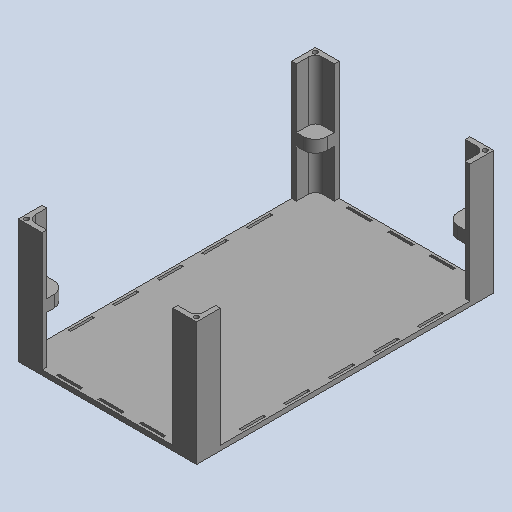
# Autodesk Inventor part: Enclosure_1
Saved by Autodesk Inventor 2026 (Build 300175050, 175E)
## iProperties
Part Number: Enclosure_1
Material: Generic
Document SubType Name: Modeling
Designer: Kartik
Mass: 216.7 g
Surface Area: 1129.54 cm^2
Volume: 216.7 cm^3
Density: 1 g/cm^3
Appearance: Default
Author: Kartik
Autodesk Inventor part; units mm, degrees
ref_plane "YZ Plane" through (0, 0, 0) normal (1, 0, 0) x (0, 1, 0)
ref_plane "XZ Plane" through (0, 0, 0) normal (0, 1, 0) x (-1, 0, 0)
ref_plane "XY Plane" through (0, 0, 0) normal (0, 0, 1) x (1, 0, 0)
sketch "Sketch1" plane through (0, 0, 0) normal (0, 1, 0) x (-1, 0, 0)
  line L0 (31.1634, 169.1828) -> (-118.8366, 169.1828)
  line L1 (-118.8366, 169.1828) -> (-118.8366, -80.8172)
  line L2 (-118.8366, -80.8172) -> (31.1634, -80.8172)
  line L3 (31.1634, -80.8172) -> (31.1634, 169.1828)
  point P0 (0, 0)
  dimension "d0" = 250
  dimension "d1" = 150
  constraints: 8 end point, 2 parallel, 1 horizontal, 1 perpendicular
  measures "d0" distance of L2.end L0.start
  measures "d1" distance of L1.end L2.end
extrude "Extrusion1" add sketch "Sketch1" along normal blind 4
fillet "Fillet1" [suppressed]
sketch "Sketch2" plane through (0, 4, 0) normal (0, 1, 0) x (1, 0, 0)
  line L0 (-31.1634, 80.8172) -> (-31.1634, -169.1828) projected
  line L1 (-31.1634, -169.1828) -> (118.8366, -169.1828) projected
  line L2 (118.8366, -169.1828) -> (118.8366, 80.8172) projected
  line L3 (118.8366, 80.8172) -> (-31.1634, 80.8172) projected
  arc A0 (-21.1634, 76.8172) -> (-27.1634, 70.8172) centre (-21.1634, 70.8172) ccw
  arc A1 (114.8366, 70.8172) -> (108.8366, 76.8172) centre (108.8366, 70.8172) ccw
  arc A2 (108.8366, -165.1828) -> (114.8366, -159.1828) centre (108.8366, -159.1828) ccw
  arc A3 (-27.1634, -159.1828) -> (-21.1634, -165.1828) centre (-21.1634, -159.1828) ccw
  line L4 (108.8366, -165.1828) -> (98.8366, -165.1828)
  line L5 (-11.1634, -165.1828) -> (-21.1634, -165.1828)
  line L6 (-27.1634, -159.1828) -> (-27.1634, -149.1828)
  line L7 (-27.1634, 60.8172) -> (-27.1634, 70.8172)
  line L8 (-21.1634, 76.8172) -> (-11.1634, 76.8172)
  line L9 (98.8366, 76.8172) -> (108.8366, 76.8172)
  line L10 (114.8366, 70.8172) -> (114.8366, 60.8172)
  line L11 (114.8366, -149.1828) -> (114.8366, -159.1828)
  line L12 (-11.1634, -169.1828) -> (-11.1634, -165.1828)
  line L13 (-11.1634, 76.8172) -> (-11.1634, 80.8172)
  line L14 (-31.1634, 60.8172) -> (-27.1634, 60.8172)
  line L15 (114.8366, 60.8172) -> (118.8366, 60.8172)
  line L16 (98.8366, -169.1828) -> (98.8366, -165.1828)
  line L17 (98.8366, 76.8172) -> (98.8366, 80.8172)
  line L18 (-31.1634, -149.1828) -> (-27.1634, -149.1828)
  line L19 (114.8366, -149.1828) -> (118.8366, -149.1828)
  point P0 (0, 0)
  point P1 (114.8366, -154.1828)
  dimension "d12" = 4
  dimension "d13" = 20
  dimension "d14" = 4
  constraints: 32 end point, 8 point on circle, 8 point on line, 4 centre point, 4 vertical, 2 horizontal, 2 perpendicular, 1 midpoint
  measures "d12" distance from line of L2 point (114.837, -154.183)
  measures "d13" distance between parallel lines of L2 L16
  measures "d14" distance between parallel lines of L2 L10
extrude "Extrusion2" add sketch "Sketch2" along normal blind 100 contours L3 L13 L8 A0 L7 L14 L0 | L18 L6 A3 L5 L12 L1 L0 | L3 L2 L15 L10 A1 L9 L17 | L16 L4 A2 L11 L19 L2 L1
sketch "Sketch3" plane through (0, 4, 0) normal (0, 1, 0) x (1, 0, 0)
  line L0 (-29.1634, -129.1828) -> (-27.1634, -129.1828)
  line L1 (-27.1634, -129.1828) -> (-27.1634, -109.1828)
  line L2 (-27.1634, -109.1828) -> (-29.1634, -109.1828)
  line L3 (-29.1634, -109.1828) -> (-29.1634, -129.1828)
  line L4 (-31.1634, 60.8172) -> (-31.1634, -149.1828) projected
  line L5 (-27.1634, -149.1828) -> (-31.1634, -149.1828) projected
  line L6 (-29.1634, -71.6828) -> (-29.1634, -91.6828)
  line L7 (-29.1634, -91.6828) -> (-27.1634, -91.6828)
  line L8 (-27.1634, -91.6828) -> (-27.1634, -71.6828)
  line L9 (-27.1634, -71.6828) -> (-29.1634, -71.6828)
  line L10 (-29.1634, -34.1828) -> (-29.1634, -54.1828)
  line L11 (-29.1634, -54.1828) -> (-27.1634, -54.1828)
  line L12 (-27.1634, -54.1828) -> (-27.1634, -34.1828)
  line L13 (-27.1634, -34.1828) -> (-29.1634, -34.1828)
  line L14 (-29.1634, 3.3172) -> (-29.1634, -16.6828)
  line L15 (-29.1634, -16.6828) -> (-27.1634, -16.6828)
  line L16 (-27.1634, -16.6828) -> (-27.1634, 3.3172)
  line L17 (-27.1634, 3.3172) -> (-29.1634, 3.3172)
  line L18 (-29.1634, 40.8172) -> (-29.1634, 20.8172)
  line L19 (-29.1634, 20.8172) -> (-27.1634, 20.8172)
  line L20 (-27.1634, 20.8172) -> (-27.1634, 40.8172)
  line L21 (-27.1634, 40.8172) -> (-29.1634, 40.8172)
  line L22 (-11.1634, -169.1828) -> (98.8366, -169.1828) projected
  line L23 (114.8366, -129.1828) -> (116.8366, -129.1828)
  line L24 (116.8366, -129.1828) -> (116.8366, -109.1828)
  line L25 (116.8366, -109.1828) -> (114.8366, -109.1828)
  line L26 (114.8366, -109.1828) -> (114.8366, -129.1828)
  line L27 (114.8366, -91.6828) -> (116.8366, -91.6828)
  line L28 (114.8366, -71.6828) -> (114.8366, -91.6828)
  line L29 (116.8366, -71.6828) -> (114.8366, -71.6828)
  line L30 (114.8366, -54.1828) -> (116.8366, -54.1828)
  line L31 (116.8366, -34.1828) -> (114.8366, -34.1828)
  line L32 (114.8366, -34.1828) -> (114.8366, -54.1828)
  line L33 (116.8366, -54.1828) -> (116.8366, -34.1828)
  line L34 (116.8366, -91.6828) -> (116.8366, -71.6828)
  line L35 (114.8366, -16.6828) -> (116.8366, -16.6828)
  line L36 (116.8366, -16.6828) -> (116.8366, 3.3172)
  line L37 (114.8366, 3.3172) -> (114.8366, -16.6828)
  line L38 (116.8366, 3.3172) -> (114.8366, 3.3172)
  line L39 (114.8366, 20.8172) -> (116.8366, 20.8172)
  line L40 (114.8366, 40.8172) -> (114.8366, 20.8172)
  line L41 (116.8366, 40.8172) -> (114.8366, 40.8172)
  line L42 (116.8366, 20.8172) -> (116.8366, 40.8172)
  line L43 (-1.1634, -167.1828) -> (18.8366, -167.1828)
  line L44 (18.8366, -167.1828) -> (18.8366, -165.1828)
  line L45 (18.8366, -165.1828) -> (-1.1634, -165.1828)
  line L46 (-1.1634, -165.1828) -> (-1.1634, -167.1828)
  line L47 (-11.1634, -169.1828) -> (-11.1634, -165.1828) projected
  line L48 (53.8366, -167.1828) -> (53.8366, -165.1828)
  line L49 (53.8366, -165.1828) -> (33.8366, -165.1828)
  line L50 (33.8366, -167.1828) -> (53.8366, -167.1828)
  line L51 (33.8366, -165.1828) -> (33.8366, -167.1828)
  line L52 (88.8366, -167.1828) -> (88.8366, -165.1828)
  line L53 (88.8366, -165.1828) -> (68.8366, -165.1828)
  line L54 (68.8366, -167.1828) -> (88.8366, -167.1828)
  line L55 (68.8366, -165.1828) -> (68.8366, -167.1828)
  line L56 (18.8366, 76.8172) -> (18.8366, 78.8172)
  line L57 (18.8366, 78.8172) -> (-1.1634, 78.8172)
  line L58 (-1.1634, 76.8172) -> (18.8366, 76.8172)
  line L59 (-1.1634, 78.8172) -> (-1.1634, 76.8172)
  line L60 (53.8366, 76.8172) -> (53.8366, 78.8172)
  line L61 (53.8366, 78.8172) -> (33.8366, 78.8172)
  line L62 (33.8366, 76.8172) -> (53.8366, 76.8172)
  line L63 (33.8366, 78.8172) -> (33.8366, 76.8172)
  line L64 (88.8366, 76.8172) -> (88.8366, 78.8172)
  line L65 (88.8366, 78.8172) -> (68.8366, 78.8172)
  line L66 (68.8366, 76.8172) -> (88.8366, 76.8172)
  line L67 (68.8366, 78.8172) -> (68.8366, 76.8172)
  point P0 (0, 0)
  point P1 (-29.1634, -149.1828)
  dimension "d15" = 2
  dimension "d16" = 20
  dimension "d17" = 2
  dimension "d18" = 20
  dimension "d21" = 37.5
  dimension "d28" = 144
  dimension "d33" = 20
  dimension "d34" = 2
  dimension "d35" = 2
  dimension "d36" = 10
  dimension "d39" = 35
  dimension "d42" = 244
  constraints: 128 end point, 4 horizontal, 4 parallel, 2 perpendicular, 2 vertical, 1 midpoint, 112 other
  measures "d15" distance of L2.end L1.end
  measures "d16" distance of L1.end L0.end
  measures "d17" distance between parallel lines of L4 L3
  measures "d18" distance from line of L0 point (-29.163, -149.183)
  measures "d21" distance of L2.end L6.start
  measures "d28" distance of L0.start L23.start
  measures "d33" distance of L45.end L44.end
  measures "d34" distance of L44.end L43.end
  measures "d35" distance between parallel lines of L22 L43
  measures "d36" distance between parallel lines of L47 L46
  measures "d39" distance of L43.end L48.start
  measures "d42" distance of L43.end L56.start
extrude "Extrusion3" cut sketch "Sketch3" against normal through all
sketch "Sketch4" plane through (0, 104, 0) normal (0, 1, 0) x (1, 0, 0)
  circle A0 centre (-27.6634, -165.6828) radius 2
  line L0 (-31.1634, -169.1828) -> (-11.1634, -169.1828) projected
  line L1 (-31.1634, -149.1828) -> (-31.1634, -169.1828) projected
  point P0 (0, 0)
  dimension "d47" = 4
  dimension "d48" = 3.5
  dimension "d49" = 3.5
  constraints: 1 centre point
  measures "d47" diameter of A0
  measures "d48" distance from line of L0 A0.centre
  measures "d49" distance from line of L1 A0.centre
extrude "Extrusion4" cut sketch "Sketch4" against normal blind 10
pattern_linear "Rectangular Pattern1" count 2 spacing 243 along (0, 0, -1) count 2 spacing 143 along (1, 0, 0) of "Extrusion4"
ref_plane "Work Plane1" through (0, 54, 0) normal (0, 1, 0) x (1, 0, 0)
sketch "Sketch5" plane through (0, 54, 0) normal (0, 1, 0) x (1, 0, 0)
  circle A0 centre (-27.6634, -165.6828) radius 2 projected
  line L0 (-27.1634, -149.1828) -> (-31.1634, -149.1828) projected
  line L1 (-31.1634, -149.1828) -> (-31.1634, -169.1828) projected
  line L2 (-31.1634, -169.1828) -> (-11.1634, -169.1828) projected
  line L3 (-11.1634, -169.1828) -> (-11.1634, -165.1828) projected
  line L4 (-11.1634, -165.1828) -> (-21.1634, -165.1828) projected
  arc A1 (-27.1634, -159.1828) -> (-21.1634, -165.1828) centre (-21.1634, -159.1828) ccw projected
  line L5 (-27.1634, -159.1828) -> (-27.1634, -149.1828) projected
  circle A2 centre (115.3366, -165.6828) radius 2 projected
  line L6 (98.8366, -165.1828) -> (98.8366, -169.1828) projected
  line L7 (98.8366, -169.1828) -> (118.8366, -169.1828) projected
  line L8 (118.8366, -169.1828) -> (118.8366, -149.1828) projected
  line L9 (118.8366, -149.1828) -> (114.8366, -149.1828) projected
  line L10 (114.8366, -149.1828) -> (114.8366, -159.1828) projected
  arc A3 (108.8366, -165.1828) -> (114.8366, -159.1828) centre (108.8366, -159.1828) ccw projected
  line L11 (108.8366, -165.1828) -> (98.8366, -165.1828) projected
  circle A4 centre (115.3366, 77.3172) radius 2 projected
  line L12 (114.8366, 60.8172) -> (118.8366, 60.8172) projected
  line L13 (118.8366, 60.8172) -> (118.8366, 80.8172) projected
  line L14 (118.8366, 80.8172) -> (98.8366, 80.8172) projected
  line L15 (98.8366, 80.8172) -> (98.8366, 76.8172) projected
  line L16 (98.8366, 76.8172) -> (108.8366, 76.8172) projected
  arc A5 (114.8366, 70.8172) -> (108.8366, 76.8172) centre (108.8366, 70.8172) ccw projected
  line L17 (114.8366, 70.8172) -> (114.8366, 60.8172) projected
  circle A6 centre (-27.6634, 77.3172) radius 2 projected
  line L18 (-11.1634, 76.8172) -> (-11.1634, 80.8172) projected
  line L19 (-11.1634, 80.8172) -> (-31.1634, 80.8172) projected
  line L20 (-31.1634, 80.8172) -> (-31.1634, 60.8172) projected
  line L21 (-31.1634, 60.8172) -> (-27.1634, 60.8172) projected
  line L22 (-27.1634, 60.8172) -> (-27.1634, 70.8172) projected
  arc A7 (-21.1634, 76.8172) -> (-27.1634, 70.8172) centre (-21.1634, 70.8172) ccw projected
  line L23 (-21.1634, 76.8172) -> (-11.1634, 76.8172) projected
  line L24 (-11.1634, -165.1828) -> (-11.1634, -149.1828)
  line L25 (-11.1634, -149.1828) -> (-27.1634, -149.1828)
  line L26 (114.8366, -149.1828) -> (98.8366, -149.1828)
  line L27 (98.8366, -149.1828) -> (98.8366, -165.1828)
  line L28 (114.8366, 60.8172) -> (98.8366, 60.8172)
  line L29 (98.8366, 60.8172) -> (98.8366, 76.8172)
  line L30 (-27.1634, 60.8172) -> (-11.1634, 60.8172)
  line L31 (-11.1634, 60.8172) -> (-11.1634, 76.8172)
  point P0 (0, 0)
  constraints: 16 end point, 5 perpendicular, 2 point on line, 1 horizontal, 1 vertical
extrude "Extrusion5" add sketch "Sketch5" against normal blind 10 contours L25 L24 L4 A1 L5 | L27 L26 L10 A3 L11 | L28 L29 L16 A5 L17 | L31 L30 L22 A7 L23
fillet "Fillet2" radius 10 4 edges at (-11.1634, 49, 149.1828) (98.8366, 49, 149.1828) (-11.1634, 49, -60.8172) (98.8366, 49, -60.8172)
body "Solid1"
